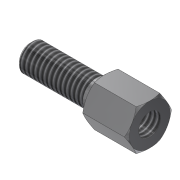
# Autodesk Inventor part: Befestigungsbolzen_M3x13-2_Provertha-531333T
Saved by Autodesk Inventor 2015 (Build 190159000, 159)
## iProperties
Created: 2015-01-30
Part Number: Befestigungsbolzen_M3x13-2_Provertha-531333T
Material: Steel
Document SubType Name: Modeling
Density: 7.85 g/cm^3
Appearance: Steel Galvanized 2
Autodesk Inventor part; units mm, degrees
ref_plane "YZ Plane" through (0, 0, 0) normal (1, 0, 0) x (0, 1, 0)
ref_plane "XZ Plane" through (0, 0, 0) normal (0, 1, 0) x (-1, 0, 0)
ref_plane "XY Plane" through (0, 0, 0) normal (0, 0, 1) x (1, 0, 0)
sketch "Sketch1" plane through (0, 0, 0) normal (1, 0, 0) x (0, 1, 0)
  line L0 (2.5981, 0) -> (1.299, -2.25)
  line L1 (1.299, -2.25) -> (-1.299, -2.25)
  line L2 (-1.299, -2.25) -> (-2.5981, 0)
  line L3 (-2.5981, 0) -> (-1.299, 2.25)
  line L4 (-1.299, 2.25) -> (1.299, 2.25)
  line L5 (1.299, 2.25) -> (2.5981, 0)
  point P0 (0, 0)
  point P1 (0, 0)
  dimension "d0" = 4.5
  constraints: 12 end point, 1 coincident, 1 horizontal alignment, 13 other
  measures "d0" distance between parallel lines of L1 L4
extrude "Extrusion1" add sketch "Sketch1" along normal blind 5
sketch "Sketch2" plane through (5, 0, 0) normal (1, 0, 0) x (0, 0, -1)
  circle A0 centre (0, 0) radius 1.5
  dimension "d3" = 3
  constraints: 1 centre point, 1 coincident
  measures "d3" diameter of A0
extrude "Extrusion2" add sketch "Sketch2" against normal blind 13.2
sketch "Sketch3" plane through (5, 0, 0) normal (1, 0, 0) x (0, 0, -1)
  point P0 (0, 0)
  point P1 (0, 0)
  constraints: 1 coincident
hole "Hole1" at (5, 0, 0) direction (-1, 0, 0) diameter 2.459 depth 4.5 tip angle 118 thread size "M3x0.5" designation "M3" class "6H" standard "ISO Metric profile"
thread "Thread1" size "M3x0.5" designation "M3" class "6g" standard "ISO Metric profile" length 7.3
chamfer "Chamfer1" distance 0.3 angle 45 1 edges at (-8.2, 0, 1.5)
sketch "Sketch4" plane through (0, 0, 0) normal (0, 1, 0) x (-1, 0, 0)
  line L0 (0, 2.25) -> (-1.7321, 5.25)
  line L1 (-1.7321, 5.25) -> (0, 5.25)
  line L2 (0, 5.25) -> (0, 2.25)
  line L3 (-3.2679, 5.25) -> (-5, 2.25)
  line L4 (-5, 2.25) -> (-5, 5.25)
  line L5 (-5, 5.25) -> (-3.2679, 5.25)
  line L6 (10.84, 0) -> (-7.64, 0) projected
  point P0 (0, 0)
  dimension "d19" = 30
  dimension "d20" = 3
  constraints: 12 end point, 2 coincident, 2 equal length, 2 perpendicular, 1 horizontal, 1 vertical
  measures "d19" angle of L2 L0
  measures "d20" distance of L1.end L0.start
revolve "Revolution1" cut sketch "Sketch4" angle 360 about axis through (-10, 0, 0) along (1, 0, 0)
body "Solid1"
